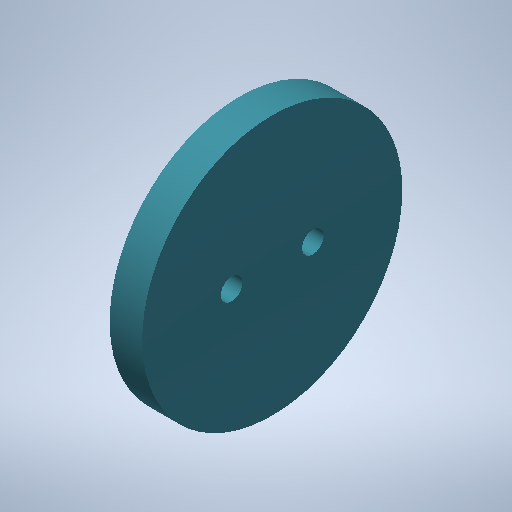
# Autodesk Inventor part: Washer
Saved by Autodesk Inventor 2025.1 (Build 291241000, 241)
## iProperties
Created: 2011-08-19
Part Number: Washer
Document SubType Name: Modeling
Designer: nguyenducthang
Density: 1 g/cm^3
Mass: 0.0230266 g
Surface Area: 0.754722 cm^2
Volume: 0.0230266 cm^3
Material: Generic
Appearance: Cadet Blue
Author: nguyenducthang
Autodesk Inventor part; units mm, degrees
ref_plane "YZ Plane" through (0, 0, 0) normal (1, 0, 0) x (0, 1, 0)
ref_plane "XZ Plane" through (0, 0, 0) normal (0, 1, 0) x (-1, 0, 0)
ref_plane "XY Plane" through (0, 0, 0) normal (0, 0, 1) x (1, 0, 0)
sketch "Sketch19" plane through (0, 0, 0) normal (1, 0, 0) x (0, 1, 0)
  circle A0 centre (0, 0) radius 12
  line L0 (0, 0) -> (12, 0) construction
  line L1 (0, 0) -> (0, 3.75) construction
  circle A1 centre (0, 3.75) radius 1
  circle A2 centre (0, -3.75) radius 1
  dimension "d111" = 24
  dimension "d112" = 2
  dimension "d113" = 3.75
  constraints: 4 end point, 2 centre point, 2 coincident, 1 horizontal, 1 horizontal alignment, 1 symmetric about line, 1 vertical, 3 other
  measures "d112" diameter of A1
  measures "d113" distance of L0.start L1.end
extrude "Extrusion16" add sketch "Sketch19" along normal blind 3
body "Solid2"
